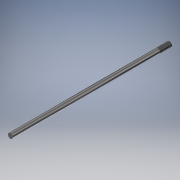
# Autodesk Inventor part: RobotArm CylinderExtension
Saved by Autodesk Inventor 2018.2 (Build 222227000, 227)
## iProperties
Created: 2018-01-15
Part Number: RobotArm CylinderExtension
Material: Generic
Document SubType Name: Modeling
Designer: lopez.xavier
Density: 1 g/cm^3
Appearance: Galvanized
Author: lopez.xavier
Autodesk Inventor part; units mm, degrees
ref_plane "YZ Plane" through (0, 0, 0) normal (1, 0, 0) x (0, 1, 0)
ref_plane "XZ Plane" through (0, 0, 0) normal (0, 1, 0) x (-1, 0, 0)
ref_plane "XY Plane" through (0, 0, 0) normal (0, 0, 1) x (1, 0, 0)
sketch "Sketch1" plane through (0, 0, 0) normal (0, 0, 1) x (1, 0, 0)
  circle A0 centre (0, 0) radius 3.175
  dimension "d0" = 6.35
  constraints: 1 centre point, 1 coincident
  measures "d0" diameter of A0
extrude "Extrusion1" add sketch "Sketch1" along normal blind 203.2
thread "Thread1" size "3/8-16 UNC" class "2A" standard "ANSI Unified Screw Threads" length 15.24 offset 187.96
body "Solid1"
